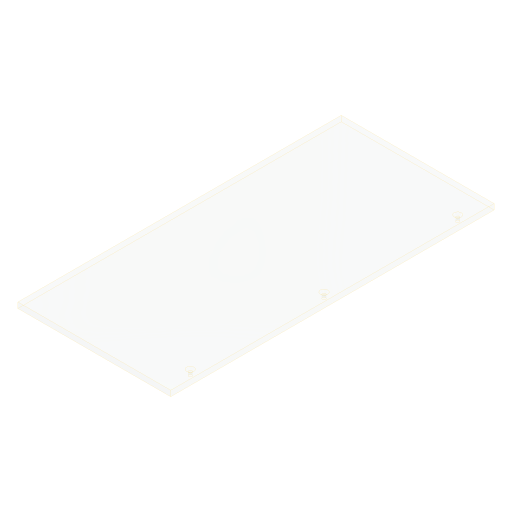
# Autodesk Inventor part: I Seitenwand
Saved by Autodesk Inventor 2023 (Build 270158000, 158)
## iProperties
Created: 2022-09-18
Part Number: I Seitenwand
Material: PVC-Piping
Document SubType Name: Modeling
Designer: musati
Density: 1.4 g/cm^3
Appearance: Oil
Author: musati
Autodesk Inventor part; units mm, degrees
ref_plane "YZ Plane" through (0, 0, 0) normal (1, 0, 0) x (0, 1, 0)
ref_plane "XZ Plane" through (0, 0, 0) normal (0, 1, 0) x (-1, 0, 0)
ref_plane "XY Plane" through (0, 0, 0) normal (0, 0, 1) x (1, 0, 0)
sketch "Skizze1" plane through (0, 0, 0) normal (0, 0, 1) x (1, 0, 0)
  line L0 (-114.8, 0) -> (114.8, 0) projected
  line L1 (0, -4.2) -> (0, 4.2) projected
  line L2 (-82, -3) -> (82, -3)
  line L3 (82, -3) -> (82, 3)
  line L4 (82, 3) -> (-82, 3)
  line L5 (-82, 3) -> (-82, -3)
  line L6 (-82, -3) -> (82, 3) construction
  line L7 (82, -3) -> (-82, 3) construction
  point P0 (0, 0)
  dimension "d0" = 164
  dimension "d1" = 6
  constraints: 12 end point, 2 midpoint, 2 parallel, 1 horizontal, 1 perpendicular
  measures "d0" distance of L4.end L3.end
  measures "d1" distance of L3.end L2.end
extrude "Extrusion1" add sketch "Skizze1" against normal blind 347
sketch "Skizze2" plane through (-82, 3, 0) normal (0, 1, 0) x (1, 0, 0)
  line L0 (164, 0) -> (0, 0) projected
  line L1 (164, 0) -> (164, 347) projected
  line L2 (0, 347) -> (164, 347) projected
  line L3 (0, 0) -> (0, 347) projected
  line L4 (-33, 0) -> (198, 0) projected
  line L5 (82, 416.4) -> (82, -69.4) projected
  point P0 (82, 0)
  point P1 (155, 30)
  point P2 (155, 173.5)
  point P3 (155, 317)
  dimension "d4" = 30
  dimension "d5" = 30
  dimension "d6" = 173.5
  dimension "d7" = 9
  dimension "d8" = 9
  dimension "d9" = 9
  measures "d4" distance from line of point (155, 30) L0
  measures "d5" distance from line of point (155, 317) L2
  measures "d6" distance from line of point (155, 173.5) L0
  measures "d7" distance from line of point (155, 30) L1
  measures "d8" distance from line of point (155, 173.5) L1
  measures "d9" distance from line of point (155, 317) L1
hole "Bohrung1" at (73, 3, -30) at (73, 3, -173.5) at (73, 3, -317) direction (0, -1, 0) diameter 3.5 depth 17 tip angle 118 countersink diameter 8 countersink angle 90
